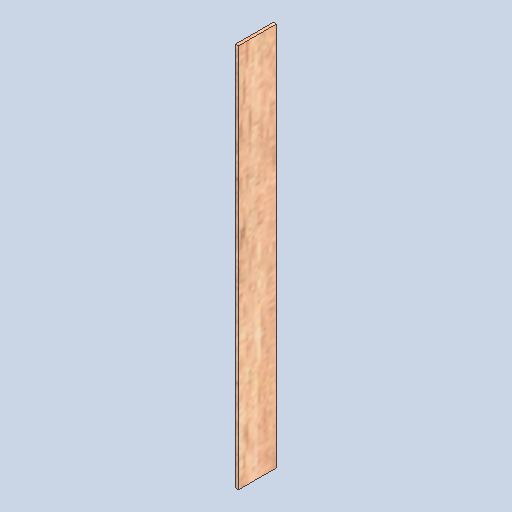
# Autodesk Inventor part: WW-01
Saved by Autodesk Inventor 2022 (Build 260153000, 153)
## iProperties
Company: El Camino Collge
Created: 2023-06-05
Part Number: WW-01
Material: Wood (Birch)
Document SubType Name: Modeling
Designer: Edgar Tejada
Density: 0.55 g/cm^3
Appearance: Birch - Natural Polished
Mass: 0.919314 g
Surface Area: 35.7935 cm^2
Volume: 1.67148 cm^3
Description: Paraffin Coated Wooden Wick
Author: Edgar Tejada
Title: Wood Wick
Autodesk Inventor part; units mm, degrees
ref_plane "YZ Plane" through (0, 0, 0) normal (1, 0, 0) x (0, 1, 0)
ref_plane "XZ Plane" through (0, 0, 0) normal (0, 1, 0) x (-1, 0, 0)
ref_plane "XY Plane" through (0, 0, 0) normal (0, 0, 1) x (1, 0, 0)
sketch "Sketch1" plane through (0, 0, 0) normal (1, 0, 0) x (0, 1, 0)
  line L0 (64.77, 6.35) -> (-64.77, 6.35)
  line L1 (-64.77, 6.35) -> (-64.77, -6.35)
  line L2 (-64.77, -6.35) -> (64.77, -6.35)
  line L3 (64.77, -6.35) -> (64.77, 6.35)
  line L4 (64.77, 6.35) -> (-64.77, -6.35) construction
  line L5 (-64.77, 6.35) -> (64.77, -6.35) construction
  point P0 (0, 0)
  dimension "d0" = 129.54
  dimension "d1" = 12.7
  constraints: 12 end point, 2 midpoint, 2 parallel, 1 horizontal, 1 perpendicular
  measures "d0" distance of L0.start L0.end
  measures "d1" distance of L2.end L0.start
extrude "Extrusion1" add sketch "Sketch1" along normal mid plane 1.016
body "Solid1"
